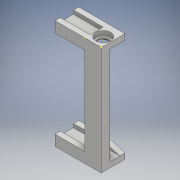
# Autodesk Inventor part: frontAxelHolder 10-23
Saved by Autodesk Inventor 2018 (Build 220112000, 112)
## iProperties
Created: 2019-10-24
Part Number: frontAxelHolder 10-23
Material: Generic
Document SubType Name: Modeling
Designer: Aditya Kendre
Density: 1 g/cm^3
Appearance: Default
Author: Aditya Kendre
Autodesk Inventor part; units mm, degrees
ref_plane "YZ Plane" through (0, 0, 0) normal (1, 0, 0) x (0, 1, 0)
ref_plane "XZ Plane" through (0, 0, 0) normal (0, 1, 0) x (-1, 0, 0)
ref_plane "XY Plane" through (0, 0, 0) normal (0, 0, 1) x (1, 0, 0)
sketch "Sketch1" plane through (0, 0, 0) normal (0, 1, 0) x (-1, 0, 0)
  line L0 (0, 0) -> (25, 0)
  line L1 (25, 0) -> (25, -165)
  line L2 (25, -165) -> (0, -165)
  line L3 (0, -165) -> (0, 0)
  dimension "d0" = 25
  dimension "d1" = 165
  constraints: 8 end point, 2 parallel, 1 horizontal, 1 perpendicular
  measures "d0" distance of L1.end L2.end
  measures "d1" distance of L0.end L1.end
extrude "Extrusion1" add sketch "Sketch1" along normal blind 3
sketch "Sketch2" plane through (0, 3, 0) normal (0, 1, 0) x (1, 0, 0)
  line L0 (0, 0) -> (0, 165) projected
  line L1 (-25, 165) -> (-25, 0) projected
  line L2 (0, 0) -> (-25, 0)
  line L3 (-25, 0) -> (-25, 8.5)
  line L4 (-25, 8.5) -> (0, 8.5)
  line L5 (0, 8.5) -> (0, 0)
  line L6 (-25, 165) -> (0, 165)
  line L7 (0, 165) -> (0, 156.5)
  line L8 (0, 156.5) -> (-25, 156.5)
  line L9 (-25, 156.5) -> (-25, 165)
  dimension "d4" = 8.5
  dimension "d5" = 8.5
  constraints: 16 end point, 4 parallel, 2 horizontal, 2 perpendicular, 2 point on line
  measures "d4" distance of L2.end L3.end
  measures "d5" distance of L6.end L7.end
extrude "Extrusion2" add sketch "Sketch2" along normal blind 25 contours L2 L1 L4 L0 | L8 L1 L6 L0
sketch "Sketch3" plane through (-25, 0, 0) normal (0, 0, 1) x (1, 0, 0)
  line L0 (0, 3) -> (0, 28) construction
  line L1 (25, 3) -> (25, 28) construction
  line L2 (0, 28) -> (25, 28) construction
  line L3 (25, 28) -> (25, 3) construction
  line L4 (25, 3) -> (0, 3) construction
  line L5 (0, 3) -> (0, 28) construction
  circle A0 centre (12.5, 15.5) radius 11
  point P0 (25, 0)
  dimension "d8" = 25
  dimension "d9" = 22
  constraints: 8 end point, 2 parallel, 1 centre point, 1 horizontal, 1 perpendicular
  measures "d8" distance of L2.end L1.start
  measures "d9" diameter of A0
extrude "Extrusion3" cut sketch "Sketch3" against normal blind 7.1
sketch "Sketch4" plane through (-25, 0, 0) normal (0, 0, 1) x (1, 0, 0)
  circle A0 centre (12.5, 15.5) radius 11 projected
  circle A1 centre (12.5, 15.5) radius 7.75
  point P0 (25, 0)
  dimension "d12" = 15.5
  constraints: 1 centre point, 1 coincident
  measures "d12" diameter of A1
extrude "Extrusion4" cut sketch "Sketch4" against normal blind 165 contours A1
sketch "Sketch5" plane through (0, 0, -165) normal (0, 0, -1) x (-1, 0, 0)
  circle A0 centre (12.5, 15.5) radius 7.75 projected
  circle A1 centre (12.5, 15.5) radius 11
  point P0 (0, 0)
  constraints: 1 centre point, 1 coincident
extrude "Extrusion5" cut sketch "Sketch5" against normal blind 7.1
sketch "Sketch6" plane through (0, 3, 0) normal (0, 1, 0) x (1, 0, 0)
  line L0 (-25, 156.5) -> (-25, 8.5) projected
  line L1 (-20.25, 8.5) -> (-4.75, 8.5) projected
  line L2 (-25, 156.5) -> (-20, 156.5)
  line L3 (-20, 156.5) -> (-20, 8.5)
  line L4 (-20, 8.5) -> (-25, 8.5)
  line L5 (-25, 8.5) -> (-25, 156.5)
  line L6 (0, 8.5) -> (0, 156.5) projected
  line L7 (-4.75, 156.5) -> (-20.25, 156.5) projected
  line L8 (0, 8.5) -> (-5, 8.5)
  line L9 (-5, 8.5) -> (-5, 156.5)
  line L10 (-5, 156.5) -> (0, 156.5)
  line L11 (0, 156.5) -> (0, 8.5)
  point P0 (0, 0)
  dimension "d17" = 5
  dimension "d18" = 5
  constraints: 16 end point, 4 parallel, 2 horizontal, 2 perpendicular, 2 point on line
  measures "d17" distance of L3.end L4.end
  measures "d18" distance of L9.end L10.end
extrude "Extrusion6" add sketch "Sketch6" along normal blind 10 contours L2 L3 L1 L4 L0 | L7 L10 L6 L8 L1 L9
fillet "Fillet1" radius 2 2 edges at (-5, 13, -82.5) (-20, 13, -82.5)
sketch "Sketch7" plane through (-25, 0, 0) normal (0, 0, 1) x (1, 0, 0)
  point P0 (25, 0)
sketch "Sketch8" plane through (-25, 0, 0) normal (0, 0, 1) x (1, 0, 0)
  circle A0 centre (12.5, 15.5) radius 11 projected
  circle A1 centre (12.5, 15.5) radius 11
  circle A2 centre (12.5, 15.5) radius 11.375
  point P0 (25, 0)
  dimension "d22" = 22.75
  constraints: 2 centre point, 2 coincident
  measures "d22" diameter of A2
extrude "Extrusion7" cut sketch "Sketch8" against normal blind 7.1
sketch "Sketch9" plane through (0, 0, -165) normal (0, 0, -1) x (-1, 0, 0)
  circle A0 centre (12.5, 15.5) radius 11.375 projected
  circle A1 centre (12.5, 15.5) radius 11.375
  point P0 (0, 0)
  constraints: 1 centre point, 1 coincident
extrude "Extrusion8" cut sketch "Sketch9" against normal blind 7.1
sketch "Sketch10" plane through (-25, 0, -165) normal (-1, 0, 0) x (0, 0, 1)
  point P0 (165, 0)
sketch "Sketch11" plane through (-25, 0, -165) normal (-1, 0, 0) x (0, 0, 1)
  line L0 (165, 0) -> (0, 0) projected
  line L1 (0, 0) -> (16, 0)
  line L2 (16, 0) -> (16, 8)
  line L3 (16, 8) -> (0, 8)
  line L4 (0, 8) -> (0, 0)
  line L5 (165, 0) -> (149, 0)
  line L6 (149, 0) -> (149, 8)
  line L7 (149, 8) -> (165, 8)
  line L8 (165, 8) -> (165, 0)
  line L9 (8.5, 28) -> (0, 28) projected
  line L10 (0, 28) -> (16, 28)
  line L11 (16, 28) -> (16, 36)
  line L12 (16, 36) -> (0, 36)
  line L13 (0, 36) -> (0, 28)
  line L14 (165, 28) -> (156.5, 28) projected
  line L15 (165, 28) -> (149, 28)
  line L16 (149, 28) -> (149, 36)
  line L17 (149, 36) -> (165, 36)
  line L18 (165, 36) -> (165, 28)
  dimension "d27" = 16
  dimension "d28" = 8
  dimension "d29" = 16
  dimension "d30" = 16
  dimension "d31" = 8
  dimension "d32" = 16
  constraints: 32 end point, 8 parallel, 4 horizontal, 4 perpendicular, 2 point on line
  measures "d27" distance of L3.end L2.end
  measures "d28" distance of L2.end L1.end
  measures "d29" distance of L6.end L7.end
  measures "d30" distance of L12.end L11.end
  measures "d31" distance of L11.end L10.end
  measures "d32" distance of L16.end L17.end
extrude "Extrusion9" add sketch "Sketch11" along normal blind 45
sketch "Sketch12" plane through (0, 28, 0) normal (0, 1, 0) x (1, 0, 0)
  line L0 (-25, 0) -> (-70, 0) projected
  line L1 (0, 0) -> (-70, 0) projected
  line L2 (-25, 0) -> (0, 0)
  line L3 (0, 0) -> (0, 8.5) projected
  line L4 (0, 0) -> (0, 8.5)
  line L5 (-25, 16) -> (-25, 0) projected
  line L6 (0, 8.5) -> (-25, 16)
  line L7 (-25, 16) -> (-25, 0)
  line L8 (-25, 16) -> (-25, 149) projected
  line L9 (0, 156.5) -> (0, 165) projected
  line L10 (-25, 149) -> (0, 156.5)
  line L11 (0, 156.5) -> (0, 165)
  line L12 (-70, 165) -> (0, 165) projected
  line L13 (0, 165) -> (-25, 165)
  line L14 (-25, 149) -> (-25, 165)
  constraints: 16 end point, 3 collinear, 1 horizontal, 1 point on line, 1 vertical
extrude "Extrusion10" add sketch "Sketch12" along normal blind 8
sketch "Sketch13" plane through (-70, 0, -165) normal (-1, 0, 0) x (0, 0, 1)
  line L0 (0, 8) -> (16, 8) construction
  line L1 (0, 0) -> (16, 0) construction
  line L2 (0, 8) -> (16, 0) construction
  line L3 (14.125, 2.25) -> (1.875, 2.25)
  line L4 (1.875, 2.25) -> (1.875, 5.75)
  line L5 (1.875, 5.75) -> (14.125, 5.75)
  line L6 (14.125, 5.75) -> (14.125, 2.25)
  line L7 (14.125, 2.25) -> (1.875, 5.75) construction
  line L8 (1.875, 2.25) -> (14.125, 5.75) construction
  line L9 (0, 0) -> (0, 36) construction
  line L10 (16, 28) -> (8.5, 28) construction
  line L11 (0, 36) -> (16, 28) construction
  line L12 (14.125, 30.25) -> (1.875, 30.25)
  line L13 (1.875, 30.25) -> (1.875, 33.75)
  line L14 (1.875, 33.75) -> (14.125, 33.75)
  line L15 (14.125, 33.75) -> (14.125, 30.25)
  line L16 (14.125, 30.25) -> (1.875, 33.75) construction
  line L17 (1.875, 30.25) -> (14.125, 33.75) construction
  line L18 (149, 0) -> (149, 8) construction
  line L19 (0, 0) -> (165, 0) construction
  line L20 (149, 8) -> (165, 0) construction
  line L21 (165, 36) -> (149, 36) construction
  line L22 (149, 28) -> (165, 28) construction
  line L23 (149, 36) -> (165, 28) construction
  line L24 (163.125, 30.25) -> (150.875, 30.25)
  line L25 (150.875, 30.25) -> (150.875, 33.75)
  line L26 (150.875, 33.75) -> (163.125, 33.75)
  line L27 (163.125, 33.75) -> (163.125, 30.25)
  line L28 (163.125, 30.25) -> (150.875, 33.75) construction
  line L29 (150.875, 30.25) -> (163.125, 33.75) construction
  line L30 (163.125, 2.25) -> (150.875, 2.25)
  line L31 (150.875, 2.25) -> (150.875, 5.75)
  line L32 (150.875, 5.75) -> (163.125, 5.75)
  line L33 (163.125, 5.75) -> (163.125, 2.25)
  line L34 (163.125, 2.25) -> (150.875, 5.75) construction
  line L35 (150.875, 2.25) -> (163.125, 5.75) construction
  point P0 (8, 4)
  point P1 (8, 32)
  point P2 (157, 32)
  point P3 (157, 4)
  dimension "d37" = 12.25
  dimension "d38" = 3.5
  dimension "d39" = 12.25
  dimension "d40" = 3.5
  dimension "d41" = 12.25
  dimension "d42" = 3.5
  dimension "d43" = 12.25
  constraints: 56 end point, 12 midpoint, 8 parallel, 4 horizontal, 4 perpendicular
  measures "d37" distance of L4.end L5.end
  measures "d38" distance of L3.end L4.end
  measures "d39" distance of L13.end L14.end
  measures "d40" distance of L12.end L13.end
  measures "d41" distance of L25.end L26.end
  measures "d42" distance of L24.end L25.end
  measures "d43" distance of L31.end L32.end
extrude "Extrusion11" cut sketch "Sketch13" against normal blind 40
sketch "Sketch14" plane through (-25, 8, -149) normal (0, 1, 0) x (1, 0, 0)
  line L0 (0, 16) -> (0, 0) construction
  line L1 (0, 8) -> (0, 10.5) construction
  line L2 (-45, 0) -> (-45, 16) projected
  line L3 (0, 10.5) -> (-45, 10.5)
  line L4 (-45, 10.5) -> (-45, 5.5)
  line L5 (-45, 5.5) -> (0, 5.5)
  line L6 (0, 5.5) -> (0, 10.5)
  line L7 (0, -133) -> (0, -149) construction
  line L8 (0, -141) -> (0, -143.5) construction
  line L9 (-45, -149) -> (-45, -133) projected
  line L10 (0, -143.5) -> (-45, -143.5)
  line L11 (-45, -143.5) -> (-45, -138.5)
  line L12 (-45, -138.5) -> (0, -138.5)
  line L13 (0, -138.5) -> (0, -143.5)
  point P0 (25, -149)
  dimension "d46" = 2.5
  dimension "d47" = 5
  dimension "d48" = 2.5
  dimension "d49" = 5
  constraints: 20 end point, 4 parallel, 4 point on line, 2 horizontal, 2 midpoint, 2 perpendicular
  measures "d46" distance of L1.start L1.end
  measures "d47" distance of L4.end L3.end
  measures "d48" distance of L8.start L8.end
  measures "d49" distance of L10.end L11.end
extrude "Extrusion12" add sketch "Sketch14" along normal blind 20
body "Solid1"
